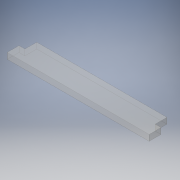
# Autodesk Inventor part: front
Saved by Autodesk Inventor 2016 (Build 200138000, 138)
## iProperties
Created: 2018-04-28
Part Number: front
Material: Polycarbonate, Clear
Document SubType Name: Modeling
Designer: Phil Erle
Density: 1.2 g/cm^3
Appearance: Polycarbonate - Clear
Author: Phil Erle
Autodesk Inventor part; units mm, degrees
ref_plane "YZ Plane" through (0, 0, 0) normal (1, 0, 0) x (0, 1, 0)
ref_plane "XZ Plane" through (0, 0, 0) normal (0, 1, 0) x (-1, 0, 0)
ref_plane "XY Plane" through (0, 0, 0) normal (0, 0, 1) x (1, 0, 0)
sketch "Sketch1" plane through (0, 0, 0) normal (0, 0, 1) x (1, 0, 0)
  line L0 (-55, 20) -> (55, 20)
  line L1 (55, 20) -> (55, 10)
  line L2 (55, 10) -> (60, 10)
  line L3 (60, 10) -> (60, 0)
  line L4 (60, 0) -> (-60, 0)
  line L5 (-60, 0) -> (-60, 10)
  line L6 (-60, 10) -> (-55, 10)
  line L7 (-55, 10) -> (-55, 20)
  point P0 (0, 0)
  point P1 (0, 20)
  dimension "d0" = 120
  dimension "d1" = 5
  dimension "d2" = 5
  dimension "d3" = 10
  dimension "d4" = 10
  constraints: 16 end point, 5 perpendicular, 2 horizontal, 2 point on line, 1 horizontal alignment, 1 midpoint, 1 vertical alignment
  measures "d0" distance of L3.end L4.end
  measures "d1" distance of L5.end L6.end
  measures "d2" distance of L1.end L2.end
  measures "d3" distance of L2.end L3.end
  measures "d4" distance of L0.end L1.end
extrude "Extrusion1" add sketch "Sketch1" along normal blind 5
body "Solid1"
